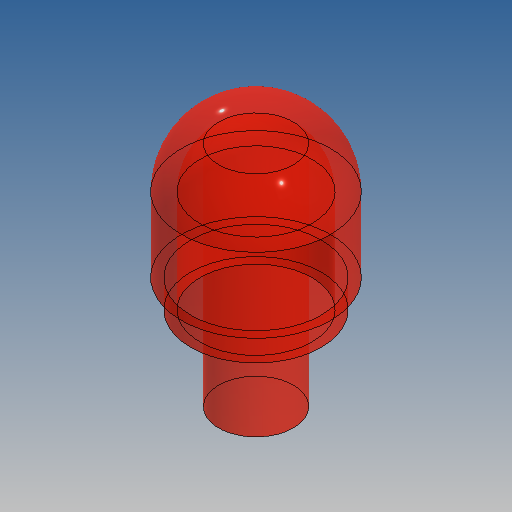
# Autodesk Inventor part: 58176-TransRed
Saved by Autodesk Inventor 2025 (Build 290162010, 162A)
## iProperties
Created: 2014-11-22
Part Number: 58176-TransRed
Material: ABS Plastic
Document SubType Name: Modeling
Designer: D. Kohfeld
Mass: 0.184291 g
Surface Area: 3.63642 cm^2
Volume: 0.173859 cm^3
Density: 1.06 g/cm^3
Appearance: TransRed
Author: D. Kohfeld
Autodesk Inventor part; units mm, degrees
ref_plane "YZ Plane" through (0, 0, 0) normal (1, 0, 0) x (0, 1, 0)
ref_plane "XZ Plane" through (0, 0, 0) normal (0, 1, 0) x (-1, 0, 0)
ref_plane "XY Plane" through (0, 0, 0) normal (0, 0, 1) x (1, 0, 0)
sketch "Sketch2" plane through (0, 0, 0) normal (0, 0, 1) x (1, 0, 0)
  line L0 (2.4, 4.4) -> (2.4, 0)
  line L1 (2.4, 0) -> (2.8, 0)
  line L2 (2.8, 0) -> (2.8, 1.2)
  line L3 (2.8, 1.2) -> (3.2, 1.2)
  line L4 (3.2, 1.2) -> (3.2, 4.4)
  arc A0 (3.2, 4.4) -> (0, 7.6) centre (0, 4.4) ccw
  line L5 (0, 7.6) -> (0, -3.6)
  line L6 (0, -3.6) -> (1.6, -3.6)
  line L7 (1.6, -3.6) -> (1.6, 6.1889)
  arc A1 (2.4, 4.4) -> (1.6, 6.1889) centre (0, 4.4) ccw
  point P0 (0, 0)
  dimension "d0" = 3.6
  dimension "d1" = 6.4
  dimension "d2" = 5.6
  dimension "d3" = 1.2
  dimension "d4" = 3.2
  dimension "d5" = 6.4
  dimension "d6" = 4.8
  constraints: 16 end point, 4 parallel, 4 point on circle, 3 perpendicular, 2 centre point, 2 point on line, 2 tangent, 1 concentric, 1 horizontal alignment, 1 vertical
  measures "d0" distance between parallel lines of L6 L1
  measures "d1" diameter of L4 L5
  measures "d2" diameter of L2 L5
  measures "d3" distance between parallel lines of L3 L1
  measures "d4" diameter of L7 L5
  measures "d5" distance from line of L5.start L3
  measures "d6" diameter of L0 L5
revolve "Revolution1" add sketch "Sketch2" angle 360 about axis through (0, 7.6, 0) along (0, -1, 0)
equation "\"d4\" = rd"
equation "\"rd\" = 3.2"
body "Solid1"
